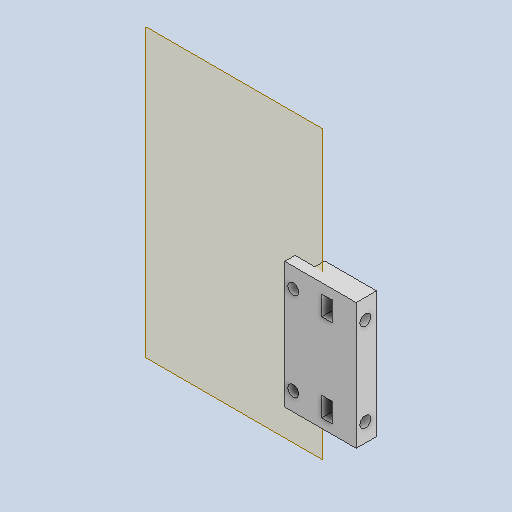
# Autodesk Inventor part: 0904_106-64_adt
Saved by Autodesk Inventor 2024.3 (Build 283343000, 343)
## iProperties
Created: 2024-09-04
Part Number: 0904_106-64_adt
Material: 일반
Document SubType Name: Modeling
Designer: gretc
Density: 1 g/cm^3
Appearance: 기본값
Author: gretc
Autodesk Inventor part; units mm, degrees
ref_plane "YZ Plane" through (0, 0, 0) normal (1, 0, 0) x (0, 1, 0)
ref_plane "XZ Plane" through (0, 0, 0) normal (0, 1, 0) x (-1, 0, 0)
ref_plane "XY Plane" through (0, 0, 0) normal (0, 0, 1) x (1, 0, 0)
ref_plane "작업 평면1" through (0, 0, 0) normal (0, 0, 1) x (1, 0, 0)
sketch "스케치1" plane through (0, 0, 0) normal (0, 0, 1) x (1, 0, 0)
  line L0 (13.5, -39.75) -> (11.5, -39.75) projected
  arc A0 (11.5, -39.75) -> (9.25, -42) centre (11.5, -42) ccw projected
  line L1 (9.25, -42) -> (9.25, -44) projected
  arc A1 (8.25, -45) -> (9.25, -44) centre (8.25, -44) ccw projected
  line L2 (8.25, -45) -> (-8.25, -45) projected
  arc A2 (-9.25, -44) -> (-8.25, -45) centre (-8.25, -44) ccw projected
  line L3 (-9.25, -44) -> (-9.25, -42) projected
  arc A3 (-9.25, -42) -> (-11.5, -39.75) centre (-11.5, -42) ccw projected
  line L4 (-11.5, -39.75) -> (-13.5, -39.75) projected
  arc A4 (-14.5, -38.75) -> (-13.5, -39.75) centre (-13.5, -38.75) ccw projected
  line L5 (-14.5, -38.75) -> (-14.5, 8.25) projected
  arc A5 (-13.5, 9.25) -> (-14.5, 8.25) centre (-13.5, 8.25) ccw projected
  line L6 (-13.5, 9.25) -> (-11.5, 9.25) projected
  arc A6 (-11.5, 9.25) -> (-9.25, 11.5) centre (-11.5, 11.5) ccw projected
  line L7 (-9.25, 11.5) -> (-9.25, 14.5) projected
  line L8 (-15, 14.5) -> (-9.25, 14.5) projected
  line L9 (-20.1, 8.5) -> (-15, 14.5) projected
  line L10 (-20.1, -44.6) -> (-20.1, 8.5) projected
  line L11 (-15, -50.6) -> (-20.1, -44.6) projected
  line L12 (15, -50.6) -> (-15, -50.6) projected
  line L13 (20.1, -44.6) -> (15, -50.6) projected
  line L14 (20.1, 8.5) -> (20.1, -44.6) projected
  line L15 (15, 14.5) -> (20.1, 8.5) projected
  line L16 (9.25, 14.5) -> (15, 14.5) projected
  line L17 (9.25, 14.5) -> (9.25, 11.5) projected
  arc A7 (9.25, 11.5) -> (11.5, 9.25) centre (11.5, 11.5) ccw projected
  line L18 (11.5, 9.25) -> (13.5, 9.25) projected
  arc A8 (14.5, 8.25) -> (13.5, 9.25) centre (13.5, 8.25) ccw projected
  line L19 (14.5, 8.25) -> (14.5, -38.75) projected
  arc A9 (13.5, -39.75) -> (14.5, -38.75) centre (13.5, -38.75) ccw projected
  circle A10 centre (17.3, 4) radius 1.35 projected
  circle A11 centre (17.3, -18) radius 1.35 projected
  circle A12 centre (11, -47.8) radius 1.35 projected
  circle A13 centre (-17.3, 4) radius 1.35 projected
  circle A14 centre (-17.3, -18) radius 1.35 projected
  circle A15 centre (-11, -47.8) radius 1.35 projected
  circle A16 centre (17.3, -40) radius 1.35 projected
  circle A17 centre (-17.3, -40) radius 1.35 projected
  line L20 (20.1, -44.6) -> (15.1755, -44.6)
  line L21 (15.1755, -44.6) -> (15.1755, -13.0737)
  line L22 (15.1755, -13.0737) -> (20.1, -13.0737)
  line L23 (20.1, -13.0737) -> (20.1, -44.6)
  point P0 (0, 0)
  point P1 (17.6377, -13.0737)
  dimension "d0" = 4.9245
  dimension "d1" = 4.9263
  constraints: 8 end point, 2 parallel, 1 horizontal, 1 midpoint, 1 perpendicular
  measures "d0" distance between parallel lines of L23 L21
  measures "d1" vertical distance of point (17.638, -13.074) A11.centre
extrude "돌출1" add sketch "스케치1" along normal blind 2.581 contours L14 L20 L21 L22
sketch "스케치6" plane through (20.1, -44.6, 0) normal (1, 0, 0) x (0, 0, -1)
  line L0 (0, 0) -> (0, 31.5263) projected
  line L1 (0, 31.5263) -> (-2.581, 31.5263) projected
  line L2 (-2.581, 0) -> (-2.581, 31.5263) projected
  line L3 (0, 0) -> (-2.581, 0) projected
  point P0 (0, 44.6)
extrude "돌출3" add sketch "스케치6" along normal blind 12.9
sketch "스케치9" plane through (0, 0, 0) normal (0, 0, -1) x (-1, 0, 0)
  line L0 (-15.1755, -44.6) -> (-33, -44.6) projected
  line L1 (-15.1755, -13.0737) -> (-15.1755, -44.6) projected
  line L2 (-15.1755, -13.0737) -> (-33, -13.0737) projected
  line L3 (-33, -44.6) -> (-33, -13.0737) projected
  circle A0 centre (-17.3, -18) radius 1.35 projected
  circle A1 centre (-17.3, -40) radius 1.35 projected
  line L4 (-20.1, 8.5) -> (-20.1, -44.6) projected
  point P0 (0, 0)
  point P1 (-20.1, -13.0737)
extrude "돌출4" add sketch "스케치9" along normal blind 2.5 contours L0 L3 L2 L4
sketch "스케치10" plane through (33, -44.6, 0) normal (1, 0, 0) x (0, 0, -1)
  circle A0 centre (-0.3, 4.6) radius 1.35 projected
  circle A1 centre (-0.3, 26.6) radius 1.35 projected
  point P0 (0, 44.6)
extrude "돌출5" cut sketch "스케치10" against normal blind 6
sketch "스케치11" plane through (0, 0, 2.581) normal (0, 0, 1) x (1, 0, 0)
  line L0 (15.1755, -44.6) -> (33, -44.6) projected
  line L1 (33, -13.0737) -> (33, -44.6) projected
  line L2 (15.1755, -13.0737) -> (33, -13.0737) projected
  line L3 (15.1755, -13.0737) -> (15.1755, -44.6) projected
  circle A0 centre (17.3, -18) radius 1.35 projected
  circle A1 centre (17.3, -40) radius 1.35 projected
  line L4 (27, -16.65) -> (27, -19.35) projected
  line L5 (27, -38.65) -> (27, -41.35) projected
  line L6 (27, -15.5189) -> (24.3972, -15.5189)
  line L7 (24.3972, -15.5189) -> (24.3972, -20.4379)
  line L8 (24.3972, -20.4379) -> (27, -20.4379)
  line L9 (27, -20.4379) -> (27, -15.5189)
  line L10 (27, -42.3162) -> (24.3972, -42.3162)
  line L11 (24.3972, -42.3162) -> (24.3972, -37.4257)
  line L12 (24.3972, -37.4257) -> (27, -37.4257)
  line L13 (27, -37.4257) -> (27, -42.3162)
  point P0 (0, 0)
  point P1 (27, -41.35)
  constraints: 16 end point, 4 parallel, 2 horizontal, 2 perpendicular
extrude "돌출6" cut sketch "스케치11" against normal blind 6 contours L4 L9 L8 L7 L6 | L5 L13 L10 L11 L12
